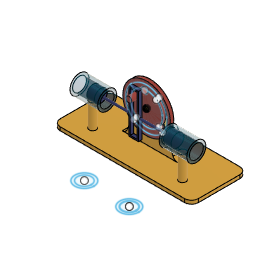
Scotch Yoke Mechanism (Autodesk Fusion 360 design; units mm, degrees)
Autodesk Fusion 360 part; units mm, degrees
note: some values were not read from the file. Chosen so that the rebuilt part matches the saved one: which face or edge a step refers to; which pieces of a blend or face edit are solid. Set by a fixed rule: which sketch regions a step uses.
sketch "suport portocaliu" plane through (0, 0, 0) normal (0, 0, 1) x (1, 0, 0) in component "suport"
  line L0 (100, -40) -> (-100, -40)
  line L1 (-100, -40) -> (-100, 40)
  line L2 (-100, 40) -> (100, 40)
  line L3 (100, 40) -> (100, -40)
  line L4 (100, -40) -> (-100, 40) construction
  line L5 (-100, -40) -> (100, 40) construction
  line L6 (0, 0) -> (35, 0)
  line L7 (35, 0) -> (35, 10)
  line L8 (35, 10) -> (0, 10)
  line L9 (0, 10) -> (0, 0)
  line L10 (0, 0) -> (-35, 0)
  line L11 (-35, 0) -> (-35, 10)
  line L12 (-35, 10) -> (0, 10)
  line L13 (0, 10) -> (0, 0)
  circle A0 centre (-85, -25) radius 6.420565
  circle A1 centre (-85, 25) radius 6.420565
  circle A2 centre (85, -25) radius 6.420565
  circle A3 centre (85, 25) radius 6.420565
  dimension "d1" = 200
  dimension "d2" = 80
  dimension "d36" = 0
  dimension "d37" = 25
  dimension "d40" = 85
  dimension "d41" = 0
  constraint horizontal L0
  constraint perpendicular L0 L1
  constraint parallel L0 L2
  constraint parallel L1 L3
  constraint coincident L4 L6.start
  constraint coincident L5 L6.start
  constraint coincident L6.start L9.end
  constraint horizontal L6
  constraint vertical L7
  constraint horizontal L8
  constraint vertical L9
  constraint horizontal L10
  constraint vertical L11
  constraint horizontal L12
  constraint vertical L13
  measures "d1" distance of L1.end L2.end
  measures "d2" distance of L0.end L1.end
extrude "Extrude1" add sketch "suport portocaliu" against normal blind 5 contours L0 L1 L2 L3 | L6 L7 L8 L9 L13 | L9 L10 L11 L12 L13 | A0 | A1 | A2 | A3 picked at (0, -20.0132) picked at (11.666667, 6.666667) picked at (-11.666667, 3.333333) picked at (-86.928243, -24.071407) picked at (-86.928243, 25.928593) picked at (83.071757, -24.071407) picked at (83.071757, 25.928593) makes body 1 in component "suport"
copy_body "CutPasteBodies1" bodies 1 removing the originals makes body 2 in component "suport"
extrude "Extrude1'" add sketch "suport portocaliu" along normal blind 65 contours L6 L7 L8 L9 L13 | L9 L10 L11 L12 L13 picked at (11.666667, 6.666667) picked at (-11.666667, 3.333333) bodies 2 in component "suport"
chamfer "Chamfer1" distance 25 distance2 65 2 edges at (-35, 5, 65) (35, 5, 65) measured on face at (11.666667, 3.333333, 65) measured on face at (11.666667, 3.333333, 65) on bodies 2 in component "suport"
fillet "Fillet1" radius 14.5 8 edges at (22.5025, 0, 32.5065) (-22.5025, 0, 32.5065) (35, 5, 0.013) (10.005, 5, 65) (22.5025, 10, 32.5065) (-10.005, 5, 65) (-35, 5, 0.013) (-22.5025, 10, 32.5065) on bodies 2 in component "suport"
fillet "Fillet2" radius 7.5 2 edges at (35, 5, 0) (-35, 5, 0) on bodies 2 in component "suport"
sketch "suport roata" plane through (0, 0, 0) normal (0, -1, 0) x (1, 0, 0) in component "suport"
  arc A0 (13.574924, 55.705197) -> (0.041413, 65) centre (0.041413, 50.5) ccw
  line L0 (0.041413, 65) -> (-0.041413, 65)
  arc A1 (-0.041413, 65) -> (-13.574924, 55.705197) centre (-0.041413, 50.5) ccw
  line L1 (-13.574924, 55.705197) -> (-33.150901, 4.807657)
  arc A2 (-40.150993, 0) -> (-33.150901, 4.807657) centre (-40.150993, 7.5) ccw
  line L2 (-40.150993, 0) -> (40.150993, 0)
  arc A3 (33.150901, 4.807657) -> (40.150993, 0) centre (40.150993, 7.5) ccw
  line L3 (33.150901, 4.807657) -> (13.574924, 55.705197)
  line L4 (0, 0) -> (-0.041413, 65)
  circle A4 centre (0.041413, 50.5) radius 2.5
  circle A5 centre (0.041413, 50.5) radius 34.288177
  dimension "d13" = 5
  constraint coincident L4.start origin
  constraint concentric A0 A4
  constraint concentric A4 A5
  measures "d13" diameter of A4
extrude "Extrude2" add sketch "suport roata" along normal blind 7 contours L4 A4 | L4 A4 picked at (0.928522, 50.930299) picked at (-1.336784, 49.969207) bodies 2 in component "suport"
fillet "Fillet3" radius 10 4 edges at (100, -40, -2.5) (100, 40, -2.5) (-100, 40, -2.5) (-100, -40, -2.5) on bodies 2 in component "suport"
extrude "Extrude1''" add sketch "suport roata" along normal blind 5 separate body contours A0 L0 L3 L4 A4 A5 | A0 L0 A1 L1 L3 A5 | A1 L1 L4 A4 A5 picked at (13.47803, 43.845509) picked at (24.219197, 63.878257) picked at (-13.403949, 43.812138) makes body 3 in component "roata"
move_face "OffsetFaces1" offset -0.3 1 faces at (-2.307818, -4.666667, 51.35505) on bodies 2 in component "suport"
sketch "modele roata" plane through (0, -5, 0) normal (0, -1, 0) x (1, 0, 0) in component "roata"
  circle A0 centre (0.041413, 50.5) radius 2.5
  circle A1 centre (0.041413, 50.5) radius 34.288177
  circle A2 centre (0.041413, 50.5) radius 29.73379
  circle A3 centre (0.041413, 50.5) radius 23.011136
  line L0 (-20.70829, 71.796669) -> (-15.991866, 67.005949)
  line L1 (-21.255255, 29.750297) -> (-16.464536, 34.466721)
  line L2 (20.791117, 29.203331) -> (16.074692, 33.994051)
  line L3 (21.338082, 71.249703) -> (16.547362, 66.533279)
  circle A4 centre (0, 72.000001) radius 4.123106
  point P0 (0.041413, 50.5)
  dimension "d22" = 360
  constraint concentric A2 A3
extrude "Extrude2'" cut sketch "modele roata" against normal blind 7 contours A2 A3 L2 L3 | A2 A3 L0 L1 picked at (20.783607, 32.539891) picked at (-20.570423, 32.403116) bodies 3 in component "roata"
fillet "Fillet1'" radius 3.5 8 edges at (16.074692, -2.5, 33.994051) (16.547362, -2.5, 66.533279) (20.791117, -2.5, 29.203331) (21.338082, -2.5, 71.249703) (-20.70829, -2.5, 71.796669) (-21.255255, -2.5, 29.750297) (-16.464536, -2.5, 34.466721) (-15.991866, -2.5, 67.005949) on bodies 3 in component "roata"
extrude "Extrude3" add sketch "modele roata" along normal blind 23 contours A3 A4 | A3 A4 picked at (-0.095618, 71.61082) picked at (-0.004539, 74.356355) bodies 3 in component "roata"
extrude "Extrude3'" add sketch "suport portocaliu" against normal blind 10 contours A0 | A1 | A2 | A3 picked at (-86.928243, -24.071407) picked at (-86.928243, 25.928593) picked at (83.071757, -24.071407) picked at (83.071757, 25.928593) bodies 2 in component "suport"
sketch "suport cilindri" plane through (0, 0, 0) normal (0, 0, 1) x (1, 0, 0) in component "cupe"
  circle A0 centre (65, -10) radius 5
  circle A1 centre (-65, -10) radius 5
  dimension "d46" = -130
  dimension "d47" = 0
extrude "Extrude1'''" add sketch "suport cilindri" along normal blind 35 separate body contours A0 | A1 picked at (64.391098, -8.448544) picked at (-66.071367, -9.525264) makes body 4 at (-60.024846, -10.497839, 23.333333) makes body 5 at (69.975154, -10.497839, 23.333333) in component "cupe"
move_body "Move1" bodies 5 to x (1, 0, 0) y (0, 1, 0) z (0, 0, 1) at (0, -6, 0) in component "cupe"
move_body "Move2" bodies 4 to x (1, 0, 0) y (0, 1, 0) z (0, 0, 1) at (0, -8, 0) in component "cupe"
move_body "Move3" bodies 5 to x (1, 0, 0) y (0, 1, 0) z (0, 0, 1) at (0, -2, 0) in component "cupe"
sketch "cilindri" plane through (0, 0, 0) normal (0, 0, 1) x (1, 0, 0) in component "cupe"
  circle A0 centre (60, -90) radius 13.730274
  circle A1 centre (60, -90) radius 10
  circle A2 centre (60, -90) radius 10
  circle A3 centre (-5, -90) radius 10
  circle A4 centre (-5, -90) radius 13.730274
  constraint concentric A0 A1
extrude "Extrude2''" add sketch "cilindri" along normal blind 40 separate body contours A0 picked at (72.3985, -91.178938) makes body 6 in component "cupe"
extrude "Extrude3''" add sketch "cilindri" along normal blind 40 separate body contours A4 picked at (7.3985, -91.178938) makes body 7 in component "cupe"
move_body "Move4" bodies 7 to x (0, 0, -1) y (0, 1, 0) z (1, 0, 0) at (-84, 72, 40.5) in component "cupe"
move_body "Move5" bodies 6 to x (0, 0, 1) y (0, 1, 0) z (-1, 0, 0) at (85, 72, -14.5) in component "cupe"
sketch "cadru" plane through (0, 0, 0) normal (0, -1, 0) x (1, 0, 0) in component "piston"
  line L0 (-5, 79.000001, 5) -> (5, 79.000001, 5)
  line L1 (5, 79.000001, 5) -> (5, 20, 5)
  line L2 (5, 20, 5) -> (-5, 20, 5)
  line L3 (-5, 20, 5) -> (-5, 79.000001, 5)
  line L4 (-7, 81.000001, 5) -> (7, 81.000001, 5)
  line L5 (7, 81.000001, 5) -> (7, 18, 5)
  line L6 (7, 18, 5) -> (-7, 18, 5)
  line L7 (-7, 18, 5) -> (-7, 81.000001, 5)
sketch "cadru (curves 5 mm off its plane)" plane through (0, -5, 0) normal (0, -1, 0) x (1, 0, 0)
  line L0 (-5, 79.000001) -> (5, 79.000001)
  line L1 (5, 79.000001) -> (5, 20)
  line L2 (5, 20) -> (-5, 20)
  line L3 (-5, 20) -> (-5, 79.000001)
  line L4 (-7, 81.000001) -> (7, 81.000001)
  line L5 (7, 81.000001) -> (7, 18)
  line L6 (7, 18) -> (-7, 18)
  line L7 (-7, 18) -> (-7, 81.000001)
extrude "Extrude1''''" add sketch "cadru (curves 5 mm off its plane)" along normal blind 5 separate body contours L4 L5 L6 L7 picked at (-6.333333, 39.666667) makes body 8 in component "piston"
move_body "Move1'" bodies 8 to x (1, 0, 0) y (0, 1, 0) z (0, 0, 1) at (0, -10, 0) in component "piston"
sketch "picior2" plane through (7, 0, 0) normal (1, 0, 0) x (0, 1, 0) in component "piston"
  line L0 (-15, 18) -> (-15, 81.000001)
  line L1 (-15, 81.000001) -> (-20, 81.000001)
  line L2 (-20, 81.000001) -> (-20, 18)
  line L3 (-20, 18) -> (-15, 18)
  circle A0 centre (-17.572139, 45.581542) radius 1.626877
extrude "Extrude2'''" add sketch "picior2" along normal blind 43 contours A0 picked at (-17.106041, 46.127694) bodies 8 in component "piston"
sketch "piston" plane through (50, 0, 0) normal (1, 0, 0) x (0, 1, 0) in component "piston"
  circle A0 centre (-17.572139, 45.581542) radius 1.626877
  circle A1 centre (-17.572139, 45.581542) radius 9.327437
  constraint concentric A0 A1
extrude "Extrude3'''" add sketch "piston" along normal blind 11 contours A1 picked at (-10.852339, 45.037323) bodies 8 in component "piston"
move_body "Move2'" bodies 8 to x (1, 0, 0) y (0, 1, 0) z (0, 0, 1) at (0, -0.1, 0) in component "piston"
sketch "picior1" plane through (-7, 0, 0) normal (-1, 0, 0) x (0, -1, 0) in component "piston"
  line L0 (15.1, 81.000001) -> (15.1, 18)
  line L1 (15.1, 18) -> (20.1, 18)
  line L2 (20.1, 18) -> (20.1, 81.000001)
  line L3 (20.1, 81.000001) -> (15.1, 81.000001)
  line L4 (17.6, 81.000001) -> (17.6, 47.208001)
  line L5 (20.1, 46.038453) -> (19.299, 46.038453)
  circle A0 centre (17.6, 45.6544) radius 1.553601
  dimension "d60" = 33.792
  dimension "d61" = 0.801
  constraint perpendicular L3 L4
  constraint perpendicular L2 L5
extrude "Extrude4" add sketch "picior1" along normal blind 43 separate body contours A0 picked at (17.747257, 46.05468) makes body 9 in component "piston"
sketch "piston1" plane through (-50, 0, 0) normal (-1, 0, 0) x (0, -1, 0) in component "piston"
  circle A0 centre (17.6, 45.6544) radius 1.553601
  circle A1 centre (17.6, 45.6544) radius 9.326597
  constraint concentric A0 A1
extrude "Extrude5" add sketch "piston1" along normal blind 11 contours A0 | A1 picked at (18.045105, 45.132847) picked at (24.295091, 45.113864) bodies 9 in component "piston"
extrude "Extrude6" add 1 faces at (50, -18.091304, 46.005523) along direction (1, 0, 0) blind 11 on bodies 8 bodies 8 in component "piston"
combine "Combine1" operation add target body 8 tool bodies 9 in component "piston"
component "suport" placed x (1, 0, 0) y (0, 1, 0) z (0, 0, 1) at (0, 0, 0)
component "roata" placed x (1, 0, 0) y (0, 1, 0) z (0, 0, 1) at (0, 0, 0)
component "cupe" placed x (1, 0, 0) y (0, 1, 0) z (0, 0, 1) at (0, 0, 0)
component "piston" placed x (1, 0, 0) y (0, 1, 0) z (0, 0, 1) at (0, 0, 0)
named bodies: "suport", "roata", "suport1", "suport2", "cilindru2", "cilindru1", "cadru"
